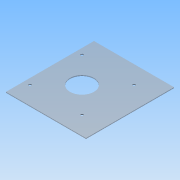
# Autodesk Inventor part: Tunel_BackCoverToOdourPort
Saved by Autodesk Inventor 2016 (Build 200138000, 138)
## iProperties
Created: 2014-11-14
Part Number: Tunel_BackCoverToOdourPort
Material: Edelstahl
Document SubType Name: Modeling
Designer: Gero Hofmann
Density: 8.08 g/cm^3
Appearance: Halbpoliert
Author: Gero Hofmann
Autodesk Inventor part; units mm, degrees
ref_plane "YZ Plane" through (0, 0, 0) normal (1, 0, 0) x (0, 1, 0)
ref_plane "XZ Plane" through (0, 0, 0) normal (0, 1, 0) x (-1, 0, 0)
ref_plane "XY Plane" through (0, 0, 0) normal (0, 0, 1) x (1, 0, 0)
sketch "Skizze1" plane through (0, 0, 0) normal (0, 0, 1) x (1, 0, 0)
  line L0 (45, -40) -> (-45, -40)
  line L1 (-45, -40) -> (-45, 40)
  line L2 (-45, 40) -> (45, 40)
  line L3 (45, 40) -> (45, -40)
  line L4 (45, -40) -> (-45, 40) construction
  line L5 (-45, -40) -> (45, 40) construction
  point P0 (0, 0)
  dimension "d0" = 90
  dimension "d1" = 80
  constraints: 12 end point, 2 midpoint, 2 parallel, 1 horizontal, 1 perpendicular
  measures "d0" distance of L1.end L2.end
  measures "d1" distance of L0.end L1.end
extrude "Extrusion1" add sketch "Skizze1" along normal blind 1
sketch "Skizze2" plane through (0, 0, 1) normal (0, 0, 1) x (1, 0, 0)
  line L0 (-45, 40) -> (-45, -40) projected
  line L1 (-45, -40) -> (45, -40) projected
  point P0 (-5, 0)
  dimension "d13" = 40
  dimension "d23" = 40
  measures "d13" distance from line of L0 point (-5, 0)
  measures "d23" distance from line of L1 point (-5, 0)
hole "Bohrung1" at (-5, 0, 1) direction (0, 0, -1) diameter 30 end through all
sketch "Skizze3" plane through (0, 0, 1) normal (0, 0, 1) x (1, 0, 0)
  circle A0 centre (-5, 0) radius 15 projected
  line L0 (30, 35) -> (-40, 35)
  line L1 (-40, 35) -> (-40, -35)
  line L2 (-40, -35) -> (30, -35)
  line L3 (30, -35) -> (30, 35)
  line L4 (30, 35) -> (-40, -35) construction
  line L5 (-40, 35) -> (30, -35) construction
  point P0 (0, 0)
  dimension "d14" = 70
  constraints: 12 end point, 3 midpoint, 2 coincident, 2 parallel, 2 perpendicular, 1 horizontal
  measures "d14" distance of L2.end L1.end
hole "Bohrung2" at (30, -35, 1) at (-40, -35, 1) at (-40, 35, 1) at (30, 35, 1) direction (0, 0, -1) diameter 4.5 end through all clearance for "Flachkopfsenkschraube DIN EN ISO 2009" size "M4" standard "DIN"
equation "\"d23\" = d13"
